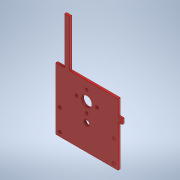
# Autodesk Inventor part: HubPlate
Saved by Autodesk Inventor 2020 (Build 240168000, 168)
## iProperties
Created: 2020-03-13
Part Number: HubPlate
Material: Generic
Document SubType Name: Modeling
Designer: jgranlund
Density: 1 g/cm^3
Appearance: Orange-Red
Author: jgranlund
Autodesk Inventor part; units mm, degrees
ref_plane "YZ Plane" through (0, 0, 0) normal (1, 0, 0) x (0, 1, 0)
ref_plane "XZ Plane" through (0, 0, 0) normal (0, 1, 0) x (-1, 0, 0)
ref_plane "XY Plane" through (0, 0, 0) normal (0, 0, 1) x (1, 0, 0)
sketch "Sketch1" plane through (0, 0, 0) normal (0, 0, 1) x (1, 0, 0)
  line L0 (0, 0) -> (-305, 0)
  line L1 (-305, 0) -> (-305, 305)
  line L2 (-305, 305) -> (-262, 305)
  line L3 (-262, 305) -> (-262, 535)
  line L4 (-262, 535) -> (-237, 535)
  line L5 (-237, 535) -> (-237, 305)
  line L6 (-237, 305) -> (0, 305)
  line L7 (0, 305) -> (0, 229)
  line L8 (0, 229) -> (20, 229)
  line L9 (20, 229) -> (20, 204)
  line L10 (20, 204) -> (0, 204)
  line L11 (0, 204) -> (0, 0)
  dimension "d0" = 305
  dimension "d1" = 305
  dimension "d4" = 230
  dimension "d5" = 25
  dimension "d6" = 230
  dimension "d7" = 76
  dimension "d8" = 20
  dimension "d9" = 25
  dimension "d10" = 43
  constraints: 24 end point, 9 perpendicular, 1 horizontal, 1 parallel, 1 point on line, 1 vertical
  measures "d0" distance of L0.start L0.end
  measures "d1" distance of L0.end L1.end
  measures "d4" distance of L2.end L3.end
  measures "d5" distance of L3.end L4.end
  measures "d6" distance of L4.end L5.end
  measures "d7" distance of L6.end L7.end
  measures "d8" distance of L7.end L8.end
  measures "d9" distance of L8.end L9.end
  measures "d10" distance of L1.end L2.end
extrude "Extrusion1" add sketch "Sketch1" along normal blind 9.5
sketch "Sketch2" plane through (0, 0, 9.5) normal (0, 0, 1) x (1, 0, 0)
  circle A0 centre (-20, 20) radius 6.5
  circle A1 centre (-20, 125) radius 6.5
  circle A2 centre (-285, 20) radius 6.5
  circle A3 centre (-285, 125) radius 6.5
  circle A4 centre (-153, 166) radius 6.25
  circle A5 centre (-153, 216) radius 25.5
  circle A6 centre (9, 216) radius 4
  line L0 (-305, 0) -> (0, 0) projected
  circle A7 centre (-103, 216) radius 6.25
  circle A8 centre (-153, 266) radius 6.25
  circle A9 centre (-203, 216) radius 6.25
  dimension "d13" = 13
  dimension "d14" = 13
  dimension "d15" = 13
  dimension "d16" = 13
  dimension "d18" = 12.5
  dimension "d21" = 8
  dimension "d22" = 20
  dimension "d23" = 20
  dimension "d24" = 20
  dimension "d25" = 20
  dimension "d26" = 125
  dimension "d27" = 20
  dimension "d28" = 20
  dimension "d29" = 125
  dimension "d30" = 216
  dimension "d31" = 216
  dimension "d32" = 166
  dimension "d35" = 360
  dimension "d37" = 51
  dimension "d38" = 103
  dimension "d39" = 162
  dimension "d40" = 162
  constraints: 10 centre point, 9 other
  measures "d13" diameter of A0
  measures "d14" diameter of A1
  measures "d15" diameter of A2
  measures "d16" diameter of A3
  measures "d18" diameter of A4
  measures "d21" diameter of A6
  measures "d22" horizontal distance of L0.end A0.centre
  measures "d23" distance from line of L0 A2.centre
  measures "d24" horizontal distance of A0.centre L0.end
  measures "d25" horizontal distance of L0.start A2.centre
  measures "d26" vertical distance of A1.centre L0.end
  measures "d27" horizontal distance of A1.centre L0.end
  measures "d28" horizontal distance of A3.centre L0.start
  measures "d29" vertical distance of A3.centre L0.start
  measures "d30" vertical distance of A6.centre L0.end
  measures "d31" vertical distance of A5.centre L0.end
  measures "d32" vertical distance of L0.end A4.centre
  measures "d37" diameter of A5
  measures "d38" horizontal distance of A7.centre L0.end
  measures "d39" distance of A5.centre A6.centre
  measures "d40" horizontal distance of A6.centre A8.centre
extrude "Extrusion2" cut sketch "Sketch2" against normal through all contours A0 | A1 | A2 | A3 | A4 | A6 | A7 | A8 | A9
sketch "Sketch3" plane through (0, 0, 9.5) normal (0, 0, 1) x (1, 0, 0)
  circle A0 centre (-203, 216) radius 6.25 projected
  circle A1 centre (-103, 216) radius 6.25 projected
  circle A2 centre (-153, 216) radius 25
  circle A3 centre (-285, 125) radius 6.5 projected
  circle A4 centre (-20, 125) radius 6.5 projected
  circle A5 centre (-153, 125) radius 12.7
  point P0 (0, 0)
  dimension "d43" = 50
  dimension "d44" = 216
  dimension "d45" = 153
  dimension "d46" = 25.4
  dimension "d47" = 125
  dimension "d48" = 153
  constraints: 2 centre point
  measures "d43" diameter of A2
  measures "d44" vertical distance of A2.centre point (0, 0)
  measures "d45" horizontal distance of A2.centre point (0, 0)
  measures "d46" diameter of A5
  measures "d47" vertical distance of A5.centre point (0, 0)
  measures "d48" horizontal distance of A5.centre point (0, 0)
extrude "Extrusion3" cut sketch "Sketch3" against normal through all contours A2 | A5
body "Solid1"
